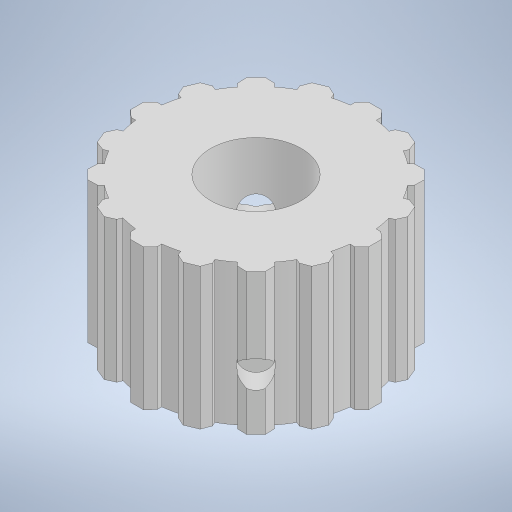
# Autodesk Inventor part: звезда_шестрерни
Saved by Autodesk Inventor 2023.1 (Build 271208000, 208)
## iProperties
Created: 2025-12-12
Part Number: звезда_шестрерни
Material: Типовые
Document SubType Name: Modeling
Designer: DELL
Density: 1 g/cm^3
Appearance: По умолчанию
Author: DELL
Autodesk Inventor part; units mm, degrees
ref_plane "YZ Plane" through (0, 0, 0) normal (1, 0, 0) x (0, 1, 0)
ref_plane "XZ Plane" through (0, 0, 0) normal (0, 1, 0) x (-1, 0, 0)
ref_plane "XY Plane" through (0, 0, 0) normal (0, 0, 1) x (1, 0, 0)
sketch "Эскиз1" plane through (0, 0, 0) normal (0, 1, 0) x (-1, 0, 0)
  line L0 (-11.15, -1.491) -> (-12.85, -1.491)
  line L1 (-13.65, -1.491) -> (-13.65, -0.741) construction
  line L2 (-13.65, 1.509) -> (-12.85, 1.509) construction
  line L3 (-11.15, 1.509) -> (-11.15, -1.491)
  circle A0 centre (0, 0) radius 12.4
  line L4 (-11.15, -1.491) -> (-13.65, 1.509) construction
  line L5 (-13.65, -1.491) -> (-11.15, 1.509) construction
  line L6 (-13.65, 0.009) -> (-11.15, 0.009) construction
  line L7 (-13.65, 0.009) -> (-13.65, 0.759)
  line L8 (-13.65, -0.741) -> (-12.85, -1.491)
  line L9 (-12.85, -1.491) -> (-12.85, 1.509) construction
  line L10 (-13.65, 0.759) -> (-12.85, 1.509)
  line L11 (-12.85, 1.509) -> (-11.15, 1.509)
  line L12 (-12.85, -1.491) -> (-13.65, -1.491) construction
  line L13 (-13.65, 0.759) -> (-13.65, 1.509) construction
  line L14 (-13.65, -0.741) -> (-13.65, 0.009)
  line L15 (-9.7307, -5.6444) -> (-11.3013, -6.295)
  line L16 (-12.0404, -6.6011) -> (-12.3274, -5.9082) construction
  line L17 (-13.1884, -3.8295) -> (-12.4493, -3.5234) construction
  line L18 (-10.8787, -2.8728) -> (-9.7307, -5.6444)
  line L19 (-9.7307, -5.6444) -> (-13.1884, -3.8295) construction
  line L20 (-12.0404, -6.6011) -> (-10.8787, -2.8728) construction
  line L21 (-12.6144, -5.2153) -> (-10.3047, -4.2586) construction
  line L22 (-12.6144, -5.2153) -> (-12.9014, -4.5224)
  line L23 (-12.3274, -5.9082) -> (-11.3013, -6.295)
  line L24 (-11.3013, -6.295) -> (-12.4493, -3.5234) construction
  line L25 (-12.9014, -4.5224) -> (-12.4493, -3.5234)
  line L26 (-12.4493, -3.5234) -> (-10.8787, -2.8728)
  line L27 (-11.3013, -6.295) -> (-12.0404, -6.6011) construction
  line L28 (-12.9014, -4.5224) -> (-13.1884, -3.8295) construction
  line L29 (-12.3274, -5.9082) -> (-12.6144, -5.2153)
  line L30 (-6.8299, -8.9385) -> (-8.032, -10.1406)
  line L31 (-8.5977, -10.7063) -> (-9.128, -10.176) construction
  line L32 (-10.719, -8.585) -> (-10.1533, -8.0193) construction
  line L33 (-8.9513, -6.8172) -> (-6.8299, -8.9385)
  line L34 (-6.8299, -8.9385) -> (-10.719, -8.585) construction
  line L35 (-8.5977, -10.7063) -> (-8.9513, -6.8172) construction
  line L36 (-9.6584, -9.6456) -> (-7.8906, -7.8779) construction
  line L37 (-9.6584, -9.6456) -> (-10.1887, -9.1153)
  line L38 (-9.128, -10.176) -> (-8.032, -10.1406)
  line L39 (-8.032, -10.1406) -> (-10.1533, -8.0193) construction
  line L40 (-10.1887, -9.1153) -> (-10.1533, -8.0193)
  line L41 (-10.1533, -8.0193) -> (-8.9513, -6.8172)
  line L42 (-8.032, -10.1406) -> (-8.5977, -10.7063) construction
  line L43 (-10.1887, -9.1153) -> (-10.719, -8.585) construction
  line L44 (-9.128, -10.176) -> (-9.6584, -9.6456)
  line L45 (-2.8894, -10.8718) -> (-3.54, -12.4424)
  line L46 (-3.8461, -13.1815) -> (-4.539, -12.8945) construction
  line L47 (-6.6178, -12.0335) -> (-6.3116, -11.2944) construction
  line L48 (-5.661, -9.7238) -> (-2.8894, -10.8718)
  line L49 (-2.8894, -10.8718) -> (-6.6178, -12.0335) construction
  line L50 (-3.8461, -13.1815) -> (-5.661, -9.7238) construction
  line L51 (-5.2319, -12.6075) -> (-4.2752, -10.2978) construction
  line L52 (-5.2319, -12.6075) -> (-5.9248, -12.3205)
  line L53 (-4.539, -12.8945) -> (-3.54, -12.4424)
  line L54 (-3.54, -12.4424) -> (-6.3116, -11.2944) construction
  line L55 (-5.9248, -12.3205) -> (-6.3116, -11.2944)
  line L56 (-6.3116, -11.2944) -> (-5.661, -9.7238)
  line L57 (-3.54, -12.4424) -> (-3.8461, -13.1815) construction
  line L58 (-5.9248, -12.3205) -> (-6.6178, -12.0335) construction
  line L59 (-4.539, -12.8945) -> (-5.2319, -12.6075)
  line L60 (1.491, -11.15) -> (1.491, -12.85)
  line L61 (1.491, -13.65) -> (0.741, -13.65) construction
  line L62 (-1.509, -13.65) -> (-1.509, -12.85) construction
  line L63 (-1.509, -11.15) -> (1.491, -11.15)
  line L64 (1.491, -11.15) -> (-1.509, -13.65) construction
  line L65 (1.491, -13.65) -> (-1.509, -11.15) construction
  line L66 (-0.009, -13.65) -> (-0.009, -11.15) construction
  line L67 (-0.009, -13.65) -> (-0.759, -13.65)
  line L68 (0.741, -13.65) -> (1.491, -12.85)
  line L69 (1.491, -12.85) -> (-1.509, -12.85) construction
  line L70 (-0.759, -13.65) -> (-1.509, -12.85)
  line L71 (-1.509, -12.85) -> (-1.509, -11.15)
  line L72 (1.491, -12.85) -> (1.491, -13.65) construction
  line L73 (-0.759, -13.65) -> (-1.509, -13.65) construction
  line L74 (0.741, -13.65) -> (-0.009, -13.65)
  line L75 (5.6444, -9.7307) -> (6.295, -11.3013)
  line L76 (6.6011, -12.0404) -> (5.9082, -12.3274) construction
  line L77 (3.8295, -13.1884) -> (3.5234, -12.4493) construction
  line L78 (2.8728, -10.8787) -> (5.6444, -9.7307)
  line L79 (5.6444, -9.7307) -> (3.8295, -13.1884) construction
  line L80 (6.6011, -12.0404) -> (2.8728, -10.8787) construction
  line L81 (5.2153, -12.6144) -> (4.2586, -10.3047) construction
  line L82 (5.2153, -12.6144) -> (4.5224, -12.9014)
  line L83 (5.9082, -12.3274) -> (6.295, -11.3013)
  line L84 (6.295, -11.3013) -> (3.5234, -12.4493) construction
  line L85 (4.5224, -12.9014) -> (3.5234, -12.4493)
  line L86 (3.5234, -12.4493) -> (2.8728, -10.8787)
  line L87 (6.295, -11.3013) -> (6.6011, -12.0404) construction
  line L88 (4.5224, -12.9014) -> (3.8295, -13.1884) construction
  line L89 (5.9082, -12.3274) -> (5.2153, -12.6144)
  line L90 (8.9385, -6.8299) -> (10.1406, -8.032)
  line L91 (10.7063, -8.5977) -> (10.176, -9.128) construction
  line L92 (8.585, -10.719) -> (8.0193, -10.1533) construction
  line L93 (6.8172, -8.9513) -> (8.9385, -6.8299)
  line L94 (8.9385, -6.8299) -> (8.585, -10.719) construction
  line L95 (10.7063, -8.5977) -> (6.8172, -8.9513) construction
  line L96 (9.6456, -9.6584) -> (7.8779, -7.8906) construction
  line L97 (9.6456, -9.6584) -> (9.1153, -10.1887)
  line L98 (10.176, -9.128) -> (10.1406, -8.032)
  line L99 (10.1406, -8.032) -> (8.0193, -10.1533) construction
  line L100 (9.1153, -10.1887) -> (8.0193, -10.1533)
  line L101 (8.0193, -10.1533) -> (6.8172, -8.9513)
  line L102 (10.1406, -8.032) -> (10.7063, -8.5977) construction
  line L103 (9.1153, -10.1887) -> (8.585, -10.719) construction
  line L104 (10.176, -9.128) -> (9.6456, -9.6584)
  line L105 (10.8718, -2.8894) -> (12.4424, -3.54)
  line L106 (13.1815, -3.8461) -> (12.8945, -4.539) construction
  line L107 (12.0335, -6.6178) -> (11.2944, -6.3116) construction
  line L108 (9.7238, -5.661) -> (10.8718, -2.8894)
  line L109 (10.8718, -2.8894) -> (12.0335, -6.6178) construction
  line L110 (13.1815, -3.8461) -> (9.7238, -5.661) construction
  line L111 (12.6075, -5.2319) -> (10.2978, -4.2752) construction
  line L112 (12.6075, -5.2319) -> (12.3205, -5.9248)
  line L113 (12.8945, -4.539) -> (12.4424, -3.54)
  line L114 (12.4424, -3.54) -> (11.2944, -6.3116) construction
  line L115 (12.3205, -5.9248) -> (11.2944, -6.3116)
  line L116 (11.2944, -6.3116) -> (9.7238, -5.661)
  line L117 (12.4424, -3.54) -> (13.1815, -3.8461) construction
  line L118 (12.3205, -5.9248) -> (12.0335, -6.6178) construction
  line L119 (12.8945, -4.539) -> (12.6075, -5.2319)
  line L120 (11.15, 1.491) -> (12.85, 1.491)
  line L121 (13.65, 1.491) -> (13.65, 0.741) construction
  line L122 (13.65, -1.509) -> (12.85, -1.509) construction
  line L123 (11.15, -1.509) -> (11.15, 1.491)
  line L124 (11.15, 1.491) -> (13.65, -1.509) construction
  line L125 (13.65, 1.491) -> (11.15, -1.509) construction
  line L126 (13.65, -0.009) -> (11.15, -0.009) construction
  line L127 (13.65, -0.009) -> (13.65, -0.759)
  line L128 (13.65, 0.741) -> (12.85, 1.491)
  line L129 (12.85, 1.491) -> (12.85, -1.509) construction
  line L130 (13.65, -0.759) -> (12.85, -1.509)
  line L131 (12.85, -1.509) -> (11.15, -1.509)
  line L132 (12.85, 1.491) -> (13.65, 1.491) construction
  line L133 (13.65, -0.759) -> (13.65, -1.509) construction
  line L134 (13.65, 0.741) -> (13.65, -0.009)
  line L135 (9.7307, 5.6444) -> (11.3013, 6.295)
  line L136 (12.0404, 6.6011) -> (12.3274, 5.9082) construction
  line L137 (13.1884, 3.8295) -> (12.4493, 3.5234) construction
  line L138 (10.8787, 2.8728) -> (9.7307, 5.6444)
  line L139 (9.7307, 5.6444) -> (13.1884, 3.8295) construction
  line L140 (12.0404, 6.6011) -> (10.8787, 2.8728) construction
  line L141 (12.6144, 5.2153) -> (10.3047, 4.2586) construction
  line L142 (12.6144, 5.2153) -> (12.9014, 4.5224)
  line L143 (12.3274, 5.9082) -> (11.3013, 6.295)
  line L144 (11.3013, 6.295) -> (12.4493, 3.5234) construction
  line L145 (12.9014, 4.5224) -> (12.4493, 3.5234)
  line L146 (12.4493, 3.5234) -> (10.8787, 2.8728)
  line L147 (11.3013, 6.295) -> (12.0404, 6.6011) construction
  line L148 (12.9014, 4.5224) -> (13.1884, 3.8295) construction
  line L149 (12.3274, 5.9082) -> (12.6144, 5.2153)
  line L150 (6.8299, 8.9385) -> (8.032, 10.1406)
  line L151 (8.5977, 10.7063) -> (9.128, 10.176) construction
  line L152 (10.719, 8.585) -> (10.1533, 8.0193) construction
  line L153 (8.9513, 6.8172) -> (6.8299, 8.9385)
  line L154 (6.8299, 8.9385) -> (10.719, 8.585) construction
  line L155 (8.5977, 10.7063) -> (8.9513, 6.8172) construction
  line L156 (9.6584, 9.6456) -> (7.8906, 7.8779) construction
  line L157 (9.6584, 9.6456) -> (10.1887, 9.1153)
  line L158 (9.128, 10.176) -> (8.032, 10.1406)
  line L159 (8.032, 10.1406) -> (10.1533, 8.0193) construction
  line L160 (10.1887, 9.1153) -> (10.1533, 8.0193)
  line L161 (10.1533, 8.0193) -> (8.9513, 6.8172)
  line L162 (8.032, 10.1406) -> (8.5977, 10.7063) construction
  line L163 (10.1887, 9.1153) -> (10.719, 8.585) construction
  line L164 (9.128, 10.176) -> (9.6584, 9.6456)
  line L165 (2.8894, 10.8718) -> (3.54, 12.4424)
  line L166 (3.8461, 13.1815) -> (4.539, 12.8945) construction
  line L167 (6.6178, 12.0335) -> (6.3116, 11.2944) construction
  line L168 (5.661, 9.7238) -> (2.8894, 10.8718)
  line L169 (2.8894, 10.8718) -> (6.6178, 12.0335) construction
  line L170 (3.8461, 13.1815) -> (5.661, 9.7238) construction
  line L171 (5.2319, 12.6075) -> (4.2752, 10.2978) construction
  line L172 (5.2319, 12.6075) -> (5.9248, 12.3205)
  line L173 (4.539, 12.8945) -> (3.54, 12.4424)
  line L174 (3.54, 12.4424) -> (6.3116, 11.2944) construction
  line L175 (5.9248, 12.3205) -> (6.3116, 11.2944)
  line L176 (6.3116, 11.2944) -> (5.661, 9.7238)
  line L177 (3.54, 12.4424) -> (3.8461, 13.1815) construction
  line L178 (5.9248, 12.3205) -> (6.6178, 12.0335) construction
  line L179 (4.539, 12.8945) -> (5.2319, 12.6075)
  line L180 (-1.491, 11.15) -> (-1.491, 12.85)
  line L181 (-1.491, 13.65) -> (-0.741, 13.65) construction
  line L182 (1.509, 13.65) -> (1.509, 12.85) construction
  line L183 (1.509, 11.15) -> (-1.491, 11.15)
  line L184 (-1.491, 11.15) -> (1.509, 13.65) construction
  line L185 (-1.491, 13.65) -> (1.509, 11.15) construction
  line L186 (0.009, 13.65) -> (0.009, 11.15) construction
  line L187 (0.009, 13.65) -> (0.759, 13.65)
  line L188 (-0.741, 13.65) -> (-1.491, 12.85)
  line L189 (-1.491, 12.85) -> (1.509, 12.85) construction
  line L190 (0.759, 13.65) -> (1.509, 12.85)
  line L191 (1.509, 12.85) -> (1.509, 11.15)
  line L192 (-1.491, 12.85) -> (-1.491, 13.65) construction
  line L193 (0.759, 13.65) -> (1.509, 13.65) construction
  line L194 (-0.741, 13.65) -> (0.009, 13.65)
  line L195 (-5.6444, 9.7307) -> (-6.295, 11.3013)
  line L196 (-6.6011, 12.0404) -> (-5.9082, 12.3274) construction
  line L197 (-3.8295, 13.1884) -> (-3.5234, 12.4493) construction
  line L198 (-2.8728, 10.8787) -> (-5.6444, 9.7307)
  line L199 (-5.6444, 9.7307) -> (-3.8295, 13.1884) construction
  line L200 (-6.6011, 12.0404) -> (-2.8728, 10.8787) construction
  line L201 (-5.2153, 12.6144) -> (-4.2586, 10.3047) construction
  line L202 (-5.2153, 12.6144) -> (-4.5224, 12.9014)
  line L203 (-5.9082, 12.3274) -> (-6.295, 11.3013)
  line L204 (-6.295, 11.3013) -> (-3.5234, 12.4493) construction
  line L205 (-4.5224, 12.9014) -> (-3.5234, 12.4493)
  line L206 (-3.5234, 12.4493) -> (-2.8728, 10.8787)
  line L207 (-6.295, 11.3013) -> (-6.6011, 12.0404) construction
  line L208 (-4.5224, 12.9014) -> (-3.8295, 13.1884) construction
  line L209 (-5.9082, 12.3274) -> (-5.2153, 12.6144)
  line L210 (-8.9385, 6.8299) -> (-10.1406, 8.032)
  line L211 (-10.7063, 8.5977) -> (-10.176, 9.128) construction
  line L212 (-8.585, 10.719) -> (-8.0193, 10.1533) construction
  line L213 (-6.8172, 8.9513) -> (-8.9385, 6.8299)
  line L214 (-8.9385, 6.8299) -> (-8.585, 10.719) construction
  line L215 (-10.7063, 8.5977) -> (-6.8172, 8.9513) construction
  line L216 (-9.6456, 9.6584) -> (-7.8779, 7.8906) construction
  line L217 (-9.6456, 9.6584) -> (-9.1153, 10.1887)
  line L218 (-10.176, 9.128) -> (-10.1406, 8.032)
  line L219 (-10.1406, 8.032) -> (-8.0193, 10.1533) construction
  line L220 (-9.1153, 10.1887) -> (-8.0193, 10.1533)
  line L221 (-8.0193, 10.1533) -> (-6.8172, 8.9513)
  line L222 (-10.1406, 8.032) -> (-10.7063, 8.5977) construction
  line L223 (-9.1153, 10.1887) -> (-8.585, 10.719) construction
  line L224 (-10.176, 9.128) -> (-9.6456, 9.6584)
  line L225 (-10.8718, 2.8894) -> (-12.4424, 3.54)
  line L226 (-13.1815, 3.8461) -> (-12.8945, 4.539) construction
  line L227 (-12.0335, 6.6178) -> (-11.2944, 6.3116) construction
  line L228 (-9.7238, 5.661) -> (-10.8718, 2.8894)
  line L229 (-10.8718, 2.8894) -> (-12.0335, 6.6178) construction
  line L230 (-13.1815, 3.8461) -> (-9.7238, 5.661) construction
  line L231 (-12.6075, 5.2319) -> (-10.2978, 4.2752) construction
  line L232 (-12.6075, 5.2319) -> (-12.3205, 5.9248)
  line L233 (-12.8945, 4.539) -> (-12.4424, 3.54)
  line L234 (-12.4424, 3.54) -> (-11.2944, 6.3116) construction
  line L235 (-12.3205, 5.9248) -> (-11.2944, 6.3116)
  line L236 (-11.2944, 6.3116) -> (-9.7238, 5.661)
  line L237 (-12.4424, 3.54) -> (-13.1815, 3.8461) construction
  line L238 (-12.3205, 5.9248) -> (-12.0335, 6.6178) construction
  line L239 (-12.8945, 4.539) -> (-12.6075, 5.2319)
  point P0 (-12.4, 0.009)
  point P1 (-11.4595, -4.737)
  point P2 (-8.7745, -8.7618)
  point P3 (-4.7536, -11.4527)
  point P4 (-0.009, -12.4)
  point P5 (4.737, -11.4595)
  point P6 (8.7618, -8.7745)
  point P7 (11.4527, -4.7536)
  point P8 (12.4, -0.009)
  point P9 (11.4595, 4.737)
  point P10 (8.7745, 8.7618)
  point P11 (4.7536, 11.4527)
  point P12 (0.009, 12.4)
  point P13 (-4.737, 11.4595)
  point P14 (-8.7618, 8.7745)
  point P15 (-11.4527, 4.7536)
  point P16 (9.7588, -7.6502)
  point P17 (10.7935, -6.1041)
  point P18 (11.9436, -3.3333)
  point P19 (12.3078, -1.509)
  point P20 (12.31, 1.491)
  point P21 (11.9484, 3.3159)
  point P22 (10.8024, 6.0884)
  point P23 (9.77, 7.6359)
  point P24 (7.6502, 9.7588)
  point P25 (6.1041, 10.7935)
  point P26 (3.3333, 11.9436)
  point P27 (1.509, 12.3078)
  point P28 (-1.491, 12.31)
  point P29 (-3.3159, 11.9484)
  point P30 (-6.0884, 10.8024)
  point P31 (-7.6359, 9.77)
  point P32 (-9.7588, 7.6502)
  point P33 (-10.7935, 6.1041)
  point P34 (-11.9436, 3.3333)
  point P35 (-12.3078, 1.509)
  point P36 (-12.31, -1.491)
  point P37 (-11.9484, -3.3159)
  point P38 (-10.8024, -6.0884)
  point P39 (-9.77, -7.6359)
  point P40 (-7.6502, -9.7588)
  point P41 (-6.1041, -10.7935)
  point P42 (-3.3333, -11.9436)
  point P43 (-1.509, -12.3078)
  point P44 (1.491, -12.31)
  point P45 (3.3159, -11.9484)
  point P46 (6.0884, -10.8024)
  point P47 (7.6359, -9.77)
  dimension "d38" = 24.8
  dimension "d0" = 2.5
  dimension "d1" = 3
  dimension "d2" = 0.8
  dimension "d5" = 360
  dimension "d36" = 136.848
  dimension "d37" = 136.848
  constraints: 480 end point, 10 perpendicular, 8 parallel, 3 midpoint, 2 horizontal, 420 other
  measures "d0" distance of L2.start L3.start
  measures "d1" distance of L1.start L2.start
  measures "d2" distance of L1.start L0.end
  measures "d36" angle of L8 L0
  measures "d37" angle of L11 L10
extrude "Выдавливание1" add sketch "Эскиз1" along normal blind 16.2
sketch "Эскиз2" plane through (10.176, 0, 9.128) normal (0.7071, 0, 0.7071) x (0.7071, 0, -0.7071)
  line L0 (-0.741, 0) -> (-0.75, 16.2) construction
  line L1 (-1.5, 16.2) -> (0, 16.2) construction
  circle A0 centre (-0.7443, 6) radius 1.6
  line L2 (-1.5, 0) -> (0, 0) projected
  dimension "d9" = 3.2
  dimension "d10" = 6
  constraints: 2 end point, 1 centre point, 1 midpoint, 1 point on line
  measures "d9" diameter of A0
  measures "d10" distance from line of L2 A0.centre
extrude "Выдавливание2" cut sketch "Эскиз2" against normal blind 10
sketch "Эскиз3" plane through (0, 0, 0) normal (0, -1, 0) x (1, 0, 0)
  line L0 (0, 0) -> (12.7279, 12.7279) construction
  line L1 (0, 0) -> (18, 0) construction
  line L2 (-1.6502, 0) -> (16.3498, 0) construction
  line L3 (4.2139, 8.103) -> (8.103, 4.2139)
  line L4 (8.103, 4.2139) -> (9.8212, 5.9322)
  line L5 (9.8212, 5.9322) -> (5.9322, 9.8212)
  line L6 (5.9322, 9.8212) -> (4.2139, 8.103)
  line L7 (4.2139, 8.103) -> (9.8212, 5.9322) construction
  line L8 (8.103, 4.2139) -> (5.9322, 9.8212) construction
  point P0 (7.0176, 7.0176)
  dimension "d14" = 45
  dimension "d17" = 5.5
  dimension "d18" = 2.43
  constraints: 18 end point, 2 horizontal, 2 midpoint, 2 parallel, 2 point on line, 1 equal length, 1 perpendicular
  measures "d14" angle of L1 L0
  measures "d17" distance of L3.start L3.end
  measures "d18" distance of L4.end L3.end
extrude "Выдавливание3" cut sketch "Эскиз3" against normal blind 9
sketch "Эскиз4" plane through (0, 0, 0) normal (0, -1, 0) x (1, 0, 0)
  circle A0 centre (0, 0) radius 5.2
  dimension "d21" = 10.4
  constraints: 1 centre point, 1 coincident
  measures "d21" diameter of A0
extrude "Выдавливание4" cut sketch "Эскиз4" against normal blind 16.2
sketch "Эскиз5" plane through (-10.176, 0, -9.128) normal (-0.7071, 0, -0.7071) x (-0.7071, 0, 0.7071)
  line L0 (-0.741, 0) -> (-0.75, 16.2) construction
  line L1 (-1.5, 16.2) -> (0, 16.2) construction
  circle A0 centre (-0.7438, 5) radius 1.6
  line L2 (-1.5, 0) -> (0, 0) projected
  line L3 (-0.7438, 5) -> (-0.746, 9)
  circle A1 centre (-0.746, 9) radius 1.6
  line L4 (-2.3264, 4.7645) -> (-2.346, 8.9926)
  line L5 (0.854, 9.0009) -> (0.8562, 5.0009)
  point P0 (-2.3285, 5.2208)
  point P1 (0.854, 9)
  dimension "d24" = 3.2
  dimension "d25" = 5
  dimension "d39" = 4
  dimension "d40" = 3.2
  constraints: 8 end point, 4 point on circle, 3 tangent, 2 centre point, 2 point on line, 1 coincident, 1 midpoint
  measures "d24" diameter of A0
  measures "d25" distance from line of L2 L3.start
  measures "d39" distance of L3.start L3.end
  measures "d40" diameter of A1
extrude "Выдавливание5" cut sketch "Эскиз5" against normal blind 10
sketch "Эскиз6" plane through (0, 0, 0) normal (0, -1, 0) x (1, 0, 0)
  circle A0 centre (0, 0) radius 8 construction
  circle A1 centre (0, 8) radius 2
  circle A2 centre (0, 0) radius 8 construction
  circle A3 centre (-8, 0) radius 2
  circle A4 centre (0, 0) radius 8 construction
  circle A5 centre (0, -8) radius 2
  circle A6 centre (0, 0) radius 8 construction
  circle A7 centre (8, 0) radius 2
  dimension "d28" = 16
  dimension "d29" = 4
  dimension "d32" = 360
  constraints: 4 centre point, 3 coincident, 2 horizontal alignment, 2 vertical alignment, 23 other
  measures "d29" diameter of A1
extrude "Выдавливание6" cut sketch "Эскиз6" against normal blind 5
